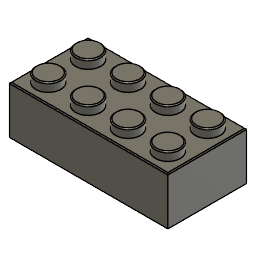
2x4 Toy Block (Autodesk Fusion 360 design; units mm, degrees)
part number: 2026-06-30-02-50-47-608
Autodesk Fusion 360 part; units mm, degrees
sketch "Sketch1" plane through (0, 0, 0) normal (0, 1, 0) x (1, 0, 0)
  line L0 (0, 0) -> (31.8, 0)
  line L1 (31.8, 0) -> (31.8, 15.8)
  line L2 (31.8, 15.8) -> (0, 15.8)
  line L3 (0, 15.8) -> (0, 0)
  dimension "d1" = 31.8
  dimension "d2" = 15.8
  constraint horizontal L0
  constraint vertical L1
  constraint horizontal L2
  constraint vertical L3
  constraint coincident L0.start L3.end
  measures "d1" distance of L0.start L0.end
  measures "d2" distance of L0.start L2.end
sketch "Sketch2" plane through (0, 0, 0) normal (0, 1, 0) x (1, 0, 0)
  line L0 (0, 0) -> (31.8, 0)
  line L1 (31.8, 0) -> (31.8, -15.8)
  line L2 (31.8, -15.8) -> (0, -15.8)
  line L3 (0, -15.8) -> (0, 0)
  dimension "d5" = 31.8
  dimension "d6" = 15.8
  constraint horizontal L0
  constraint vertical L1
  constraint horizontal L2
  constraint vertical L3
  constraint coincident L0.start L3.end
  measures "d5" distance of L0.start L0.end
  measures "d6" distance of L0.start L2.end
extrude "Extrude2" add sketch "Sketch2" along normal blind 9.6
sketch "Sketch3" plane through (0, 9.6, 0) normal (0, 1, 0) x (-1, 0, 0)
  line L0 (0, 15.8) -> (-31.8, 15.8)
  line L1 (-31.8, 15.8) -> (-31.8, 0)
  line L2 (-31.8, 0) -> (0, 0)
  line L3 (0, 0) -> (0, 15.8)
  circle A0 centre (-3.9, 3.9) radius 2.5
  dimension "d9" = 5
  dimension "d10" = 3.9
  dimension "d11" = 3.9
  measures "d9" diameter of A0
  measures "d10" distance of L2 A0.centre
  measures "d11" distance of L3 A0.centre
extrude "Extrude3" add sketch "Sketch3" along normal blind 1.7 contours A0
pattern_linear "R-Pattern1" count 4 spacing 8 along (1, 0, 0) count 2 spacing 8 along (0, 0, 1) of "Extrude3"
shell "Shell1" thickness 1.49 removed faces 1 at (10.6, 0, 10.5333)
sketch "Sketch4" plane through (0, 8.11, 0) normal (0, -1, 0) x (1, 0, 0)
  line L0 (30.31, 14.31) -> (1.49, 14.31)
  line L1 (1.49, 14.31) -> (1.49, 1.49)
  line L2 (1.49, 1.49) -> (30.31, 1.49)
  line L3 (30.31, 1.49) -> (30.31, 14.31)
  circle A0 centre (3.9, 3.9) radius 1.01
  circle A1 centre (11.9, 3.9) radius 1.01
  circle A2 centre (19.9, 3.9) radius 1.01
  circle A3 centre (27.9, 3.9) radius 1.01
  circle A4 centre (3.9, 11.9) radius 1.01
  circle A5 centre (11.9, 11.9) radius 1.01
  circle A6 centre (19.9, 11.9) radius 1.01
  circle A7 centre (27.9, 11.9) radius 1.01
  line L4 (3.9, 11.9) -> (11.9, 3.9) construction
  circle A8 centre (7.9, 7.9) radius 3.15
  circle A9 centre (7.9, 7.9) radius 2.15
  dimension "d19" = 6.3
  dimension "d20" = -1
  constraint coincident A4.centre L4.start
  constraint coincident A1.centre L4.end
  constraint midpoint L4 A8.centre
  measures "d19" diameter of A8
extrude "Extrude4" add sketch "Sketch4" along normal blind 8.1 contours A8
pattern_linear "R-Pattern2" count 3 spacing 8 along (1, 0, 0) of "Extrude4"
fillet "Fillet1" radius 0.2 15 edges at (6.2308, 11.3, 10.996) (6.2308, 11.3, 2.996) (14.2308, 11.3, 10.996) (14.2308, 11.3, 2.996) (22.2308, 11.3, 10.996) (22.2308, 11.3, 2.996) (30.2308, 11.3, 10.996) (30.2308, 11.3, 2.996) (15.9, 9.6, 0) (0, 9.6, 7.9) (15.9, 9.6, 15.8) (31.8, 9.6, 7.9) (20.9632, 0.01, 6.7609) (12.9632, 0.01, 6.7609) (4.9632, 0.01, 6.7609)
